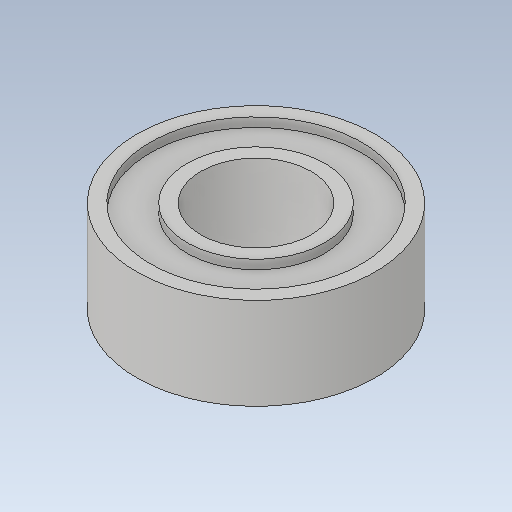
# Autodesk Inventor part: bearing_6_13_5
Saved by Autodesk Inventor 2020 (Build 240168000, 168)
## iProperties
Part Number: bearing_6_13_5
Material: 常规
Document SubType Name: Modeling
Designer: psrob
Density: 1 g/cm^3
Appearance: 默认
Mass: 0.358142 g
Surface Area: 5.07367 cm^2
Volume: 0.358142 cm^3
Author: psrob
Autodesk Inventor part; units mm, degrees
ref_plane "YZ Plane" through (0, 0, 0) normal (1, 0, 0) x (0, 1, 0)
ref_plane "XZ Plane" through (0, 0, 0) normal (0, 1, 0) x (-1, 0, 0)
ref_plane "XY Plane" through (0, 0, 0) normal (0, 0, 1) x (1, 0, 0)
sketch "草图1" plane through (0, 0, 0) normal (0, 1, 0) x (-1, 0, 0)
  circle A0 centre (0, 0) radius 6.5
  circle A1 centre (0, 0) radius 3
  dimension "d0" = 13
  dimension "d1" = 6
  constraints: 2 centre point, 2 coincident
  measures "d0" diameter of A0
  measures "d1" diameter of A1
extrude "拉伸1" add sketch "草图1" along normal blind 5
sketch "草图2" plane through (0, 5, 0) normal (0, 1, 0) x (1, 0, 0)
  circle A0 centre (0, 0) radius 3 projected
  circle A1 centre (0, 0) radius 6.5 projected
  circle A2 centre (0, 0) radius 3.75
  circle A3 centre (0, 0) radius 5.75
  dimension "d4" = 11.5
  dimension "d5" = 7.5
  constraints: 2 centre point, 2 coincident
  measures "d4" diameter of A3
  measures "d5" diameter of A2
extrude "拉伸2" cut sketch "草图2" against normal blind 0.5 contours A3
sketch "草图3" plane through (0, 0, 0) normal (0, -1, 0) x (1, 0, 0)
  circle A0 centre (0, 0) radius 3.75 projected
  circle A1 centre (0, 0) radius 5.75 projected
extrude "拉伸3" cut sketch "草图3" against normal blind 0.5
